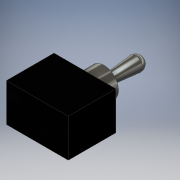
# Autodesk Inventor part: toggle switch
Saved by Autodesk Inventor 2016 (Build 200138000, 138)
## iProperties
Created: 2016-05-17
Part Number: toggle switch
Material: Generic
Document SubType Name: Modeling
Designer: Lillahunden
Density: 1 g/cm^3
Appearance: Default
Author: Lillahunden
Autodesk Inventor part; units mm, degrees
ref_plane "YZ Plane" through (0, 0, 0) normal (1, 0, 0) x (0, 1, 0)
ref_plane "XZ Plane" through (0, 0, 0) normal (0, 1, 0) x (-1, 0, 0)
ref_plane "XY Plane" through (0, 0, 0) normal (0, 0, 1) x (1, 0, 0)
sketch "Sketch1" plane through (0, 0, 0) normal (0, 1, 0) x (-1, 0, 0)
  circle A0 centre (0, 0) radius 3.05
  dimension "d0" = 6.1
  constraints: 1 centre point, 1 coincident
  measures "d0" diameter of A0
extrude "Extrusion1" add sketch "Sketch1" along normal blind 4
sketch "Sketch2" plane through (0, 0, 0) normal (1, 0, 0) x (0, 1, 0)
  line L0 (12.1205, 0) -> (4, 0)
  line L1 (4, -3.05) -> (4, 3.05) projected
  arc A0 (10.3569, -1.4766) -> (12.1205, 0) centre (10.6205, 0) ccw
  line L2 (4, -0.9136) -> (10.6205, -1.5)
  line L3 (4, -0.9136) -> (4, 0)
  point P0 (0, 0)
  dimension "d3" = 3
  constraints: 6 end point, 3 point on circle, 3 point on line, 1 centre point, 1 collinear, 1 midpoint
  measures "d3" diameter of A0
revolve "Revolution1" add sketch "Sketch2" angle 360 about axis through (0, 12.1205, 0) along (0, -1, 0) contours A0 L2 L1 L0
sketch "Sketch3" plane through (0, 0, 0) normal (0, -1, 0) x (1, 0, 0)
  line L0 (6.5, 4) -> (-6.5, 4)
  line L1 (-6.5, 4) -> (-6.5, -4)
  line L2 (-6.5, -4) -> (6.5, -4)
  line L3 (6.5, -4) -> (6.5, 4)
  point P0 (0, 0)
  point P1 (-6.5, 0)
  point P2 (0, 4)
  dimension "d5" = 13
  dimension "d6" = 8
  constraints: 8 end point, 2 midpoint, 2 parallel, 1 horizontal, 1 horizontal alignment, 1 perpendicular, 1 vertical alignment
  measures "d5" distance of L2.end L1.end
  measures "d6" distance of L1.end L0.end
extrude "Extrusion2" add sketch "Sketch3" along normal blind 10
body "Solid1"
